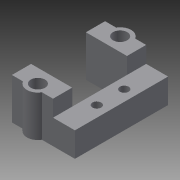
# Autodesk Inventor part: servo_holder
Saved by Autodesk Inventor 2015 (Build 190159000, 159)
## iProperties
Created: 2017-12-08
Part Number: servo_holder
Material: Generic
Document SubType Name: Modeling
Designer: Anshul
Density: 1 g/cm^3
Appearance: Default
Author: Anshul
Autodesk Inventor part; units mm, degrees
ref_plane "YZ Plane" through (0, 0, 0) normal (1, 0, 0) x (0, 1, 0)
ref_plane "XZ Plane" through (0, 0, 0) normal (0, 1, 0) x (-1, 0, 0)
ref_plane "XY Plane" through (0, 0, 0) normal (0, 0, 1) x (1, 0, 0)
sketch "Sketch1" plane through (0, 0, 0) normal (0, 1, 0) x (-1, 0, 0)
  line L0 (0, 0) -> (0, -34)
  line L1 (0, -34) -> (8, -34)
  line L2 (8, -34) -> (8, 0)
  line L3 (8, 0) -> (0, 0)
  line L4 (23, -34) -> (23, -27)
  line L5 (23, -27) -> (8, -27)
  line L6 (23, 0) -> (23, -7)
  line L7 (23, -7) -> (8, -7)
  line L8 (8, -7) -> (8, -27)
  line L9 (8, -17) -> (4, -17)
  line L10 (4, -17) -> (4, -22)
  line L11 (4, -17) -> (4, -12)
  circle A0 centre (4, -12) radius 1.6
  circle A1 centre (4, -22) radius 1.6
  line L12 (8, -7) -> (0, -7)
  line L13 (8, -27) -> (0, -27)
  line L14 (23, -7) -> (23, -2)
  circle A2 centre (15.5, -2) radius 2.6
  arc A3 (18.9641, 0) -> (12.0359, 0) centre (15.5, -2) ccw
  line L15 (8, 0) -> (12.0359, 0)
  line L16 (18.9641, 0) -> (23, 0)
  line L17 (23, -27) -> (23, -32)
  circle A4 centre (15.5, -32) radius 2.6
  arc A5 (12.0359, -34) -> (18.9641, -34) centre (15.5, -32) ccw
  line L18 (8, -34) -> (12.0359, -34)
  line L19 (18.9641, -34) -> (23, -34)
  circle A6 centre (4, -12) radius 3
  circle A7 centre (4, -22) radius 3
  dimension "d0" = 34
  dimension "d1" = 8
  dimension "d2" = 15
  dimension "d3" = 7
  dimension "d4" = 15
  dimension "d5" = 7
  dimension "d6" = 4
  dimension "d7" = 5
  dimension "d8" = 5
  dimension "d9" = 3.2
  dimension "d10" = 3.2
  dimension "d11" = 5
  dimension "d12" = 5.2
  dimension "d13" = 8
  dimension "d14" = 5
  dimension "d15" = 5.2
  dimension "d16" = 8
  dimension "d21" = 6
  dimension "d22" = 6
  constraints: 40 end point, 10 point on line, 8 centre point, 8 perpendicular, 6 coincident, 4 point on circle, 2 horizontal, 2 vertical, 1 collinear, 1 midpoint
  measures "d0" distance of L0.start L0.end
  measures "d1" distance of L0.end L1.end
  measures "d2" distance of L1.end L4.start
  measures "d3" distance of L4.start L4.end
  measures "d4" distance of L2.end L6.start
  measures "d5" distance of L6.start L6.end
  measures "d6" distance of L9.start L9.end
  measures "d7" distance of L9.end L10.end
  measures "d8" distance of L9.end L11.end
  measures "d9" diameter of A0
  measures "d10" diameter of A1
  measures "d11" distance of L6.end L14.end
  measures "d12" diameter of A2
  measures "d13" diameter of A3
  measures "d14" distance of L4.end L17.end
  measures "d15" diameter of A4
  measures "d16" diameter of A5
  measures "d21" diameter of A6
  measures "d22" diameter of A7
extrude "Extrusion1" add sketch "Sketch1" along normal blind 9 contours L3 L2 L12 L0 | L12 L2 L13 L0 | L13 L2 L1 L0 | A6 | A7
extrude "Extrusion2" add sketch "Sketch1" along normal blind 15 contours L15 A3 L16 L6 L7 L2 | L5 L4 L19 A5 L18 L2
extrude "Extrusion3" cut sketch "Sketch1" along normal blind 4 contours A6 | A7
fillet "Fillet1" radius 2 2 edges at (-1, 4, -22) (-1, 4, -12)
body "Solid1"
